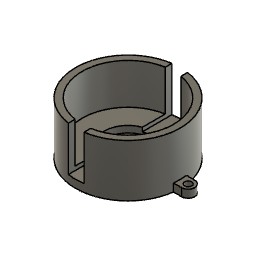
Motorholder v3 (Autodesk Fusion 360 design; units mm, degrees)
Autodesk Fusion 360 part; units mm, degrees
sketch "Sketch2" plane through (0, 0, 0) normal (0, 0, 1) x (1, 0, 0)
  line L0 (0, -19) -> (0, -17)
  line L1 (0, -17) -> (0, 22) construction
  line L2 (-22, 0) -> (25, 0) construction
  line L3 (0, 0) -> (5, 0)
  line L4 (20, 0) -> (20, 20)
  line L5 (0, 0) -> (20, 0)
  line L6 (20, 20) -> (17.5, 20)
  line L7 (17.5, 20) -> (17.5, 4.5)
  line L8 (17.5, 4.5) -> (9, 4.5)
  line L9 (9, 4.5) -> (9, 2)
  line L10 (9, 2) -> (0, 2)
  line L11 (0, 2) -> (0, 0)
  dimension "d76" = 20
  dimension "d77" = 20
  dimension "d78" = 2
  dimension "d79" = 4.5
  dimension "d80" = 17.5
  dimension "d81" = 9
  constraint vertical L0
  constraint parallel L0 L1
  constraint horizontal L2
  constraint coincident L3.start L5.start
  constraint coincident L2 L3.end
  constraint perpendicular L1 L3
  constraint coincident L2 L4.start
  constraint perpendicular L2 L4
  constraint perpendicular L4 L6
  constraint perpendicular L6 L7
  constraint perpendicular L4 L8
  constraint perpendicular L8 L9
  constraint coincident L1 L10.end
  constraint perpendicular L1 L10
  measures "d76" distance of L1 L4
  measures "d77" distance of L2 L6
  measures "d78" distance of L5 L10
  measures "d79" distance of L2 L8.end
  measures "d80" distance of L1 L7
  measures "d81" distance of L1 L9
revolve "Revolve1" add sketch "Sketch2" angle 360 about axis through (0, -17, 0) along (0, 1, 0)
sketch "Sketch3" plane through (0, 0, 0) normal (0, -1, 0) x (1, 0, 0)
  circle A0 centre (0, 0) radius 20
  line L0 (3, -19.7737) -> (3, 19.7737)
  circle A1 centre (0, 0) radius 20
  line L1 (0, 1.75) -> (0, 22.5)
  line L2 (-3, -19.7737) -> (-3, 19.7737)
  line L3 (-19.8431, 2.5) -> (-23, 2.5)
  arc A2 (-23, 2.5) -> (-23, -2.5) centre (-23, 0) ccw
  line L4 (-23, -2.5) -> (-19.8431, -2.5)
  line L5 (-15, 0) -> (-23, 0) construction
  arc A3 (23, -2.5) -> (23, 2.5) centre (23, 0) ccw
  line L6 (23, -2.5) -> (19.8431, -2.5)
  line L7 (15, 0) -> (23, 0) construction
  line L8 (19.8431, 2.5) -> (23, 2.5)
  circle A4 centre (-23, 0) radius 1.375
  circle A5 centre (23, 0) radius 1.375
  dimension "d83" = 6
  dimension "d84" = 5
  dimension "d88" = 2.75
  constraint vertical L0
  constraint coincident A0 L0.end
  constraint coincident A0 L0.start
  constraint symmetric L0.end L1 L2.end
  constraint symmetric L0.start L1 L2.start
  constraint tangent L3 A2
  constraint tangent A2 L4
  constraint parallel L3 L4
  constraint horizontal L5
  constraint coincident A0 L3.start
  constraint coincident A0 L4.end
  constraint symmetric L1 L3.end A3.end
  constraint symmetric L1 A2.end A3.start
  constraint symmetric L1 L5.start L7.start
  constraint symmetric L1 A2 A3
  constraint symmetric L1 L3.start L8.start
  constraint symmetric L1 L4.end L6.end
  constraint concentric A2 A4
  constraint symmetric L1 A4 A5
  measures "d83" distance of L0 L2
  measures "d84" diameter of A2
  measures "d88" diameter of A4
extrude "Extrude4" cut sketch "Sketch3" against normal blind 17 from surface at -3 contours A0 L0 A1 L2
extrude "Extrude5" add sketch "Sketch3" against normal blind 3 contours A0 A1 A3 L6 L8 | A0 A1 L3 A2 L4
sketch "Sketch4" plane through (0, 0, 0) normal (0, 0, 1) x (1, 0, 0)
named bodies: "holder"
